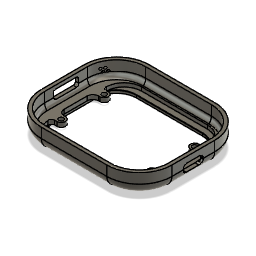
cube2025年6月14日 (Autodesk Fusion 360 design; units mm, degrees)
Autodesk Fusion 360 part; units mm, degrees
sketch "草图1" plane through (0, 0, 0) normal (0, 1, 0) x (1, 0, 0)
  line L0 (11.6, 15.075) -> (-11.6, 15.075)
  line L1 (-19.1, 7.575) -> (-19.1, -7.575)
  line L2 (-11.6, -15.075) -> (11.6, -15.075)
  line L3 (19.1, -7.575) -> (19.1, 7.575)
  line L4 (19.1, 15.075) -> (-19.1, -15.075) construction
  line L5 (-19.1, 15.075) -> (19.1, -15.075) construction
  arc A0 (-11.6, 15.075) -> (-19.1, 7.575) centre (-11.6, 7.575) ccw
  arc A1 (19.1, 7.575) -> (11.6, 15.075) centre (11.6, 7.575) ccw
  arc A2 (11.6, -15.075) -> (19.1, -7.575) centre (11.6, -7.575) ccw
  arc A3 (-19.1, -7.575) -> (-11.6, -15.075) centre (-11.6, -7.575) ccw
  dimension "d1" = 38.2
  dimension "d2" = 30.15
  dimension "d3" = 7.5
  dimension "d4" = 7.5
  constraint horizontal L0
  constraint perpendicular L0 L1
  constraint parallel L0 L2
  constraint parallel L1 L3
  constraint coincident L4 origin
  constraint coincident L5 origin
  constraint coincident L5.start L1
  constraint coincident L5.start L0
  constraint tangent L1 A0
  constraint tangent L0 A0
  constraint coincident L4.start L0
  constraint coincident L4.start L3
  constraint tangent L0 A1
  constraint tangent L3 A1
  constraint coincident L5.end L3
  constraint coincident L5.end L2
  constraint tangent L3 A2
  constraint tangent L2 A2
  constraint equal A1 A2
  constraint coincident L4.end L1
  constraint coincident L4.end L2
  constraint tangent L1 A3
  constraint tangent L2 A3
  constraint equal A1 A3
  measures "d1" distance of L4.end L5.end
  measures "d2" distance of L4.start L5.end
  measures "d3" radius of A0
  measures "d4" radius of A1
sketch "草图2" plane through (0, 0, 0) normal (0, 1, 0) x (1, 0, 0)
  circle A0 centre (17.3934, 13.5745) radius 0.65
  circle A1 centre (-17.3935, -13.5745) radius 0.65
  circle A2 centre (17.3934, -13.5745) radius 0.65
  circle A3 centre (-17.3935, 13.5745) radius 0.65
  arc A4 (-16.0995, 15.5745) -> (-19.3935, 12.4745) centre (-16.0995, 12.2745) ccw
  arc A5 (-19.3935, -12.4745) -> (-16.0995, -15.5745) centre (-16.0995, -12.2745) ccw
  arc A6 (16.0995, -15.5745) -> (19.3934, -12.4745) centre (16.0995, -12.2745) ccw
  line L0 (-16.0995, -15.5745) -> (16.0995, -15.5745)
  line L1 (19.3934, -12.4745) -> (19.3934, 12.4745)
  arc A7 (19.3934, 12.4745) -> (16.0995, 15.5745) centre (16.0995, 12.2745) ccw
  line L2 (-19.3935, 12.4745) -> (-19.3935, -12.4745)
  line L3 (16.0995, 15.5745) -> (-16.0995, 15.5745)
  line L4 (-17.3935, 13.5745) -> (17.3934, -13.5745)
  line L5 (17.3934, 13.5745) -> (-17.3935, -13.5745)
sketch "草图3" plane through (0, 0, 0) normal (0, 0, 1) x (1, 0, 0)
  line L0 (0, 0) -> (19.1, 0)
  line L1 (0, 0) -> (-19.1, 0)
  line L2 (0, 0) -> (0, 4.5)
  line L3 (0, 4.5) -> (23.1, 4.5)
  line L4 (0, 4.5) -> (-23.1, 4.5)
  line L5 (19.1, 0) -> (19.4, 0)
  line L6 (19.4, 0) -> (19.4, 0.5)
  line L7 (19.4, 0.5) -> (19.1, 0.5)
  line L8 (19.1, 0.5) -> (19.1, 0)
  line L9 (-19.1, 0) -> (-19.4, 0)
  line L10 (-19.4, 0) -> (-19.4, 0.5)
  line L11 (-19.4, 0.5) -> (-19.1, 0.5)
  line L12 (-19.1, 0.5) -> (-19.1, 0)
  circle A0 centre (19.1, 4.5) radius 4
  circle A1 centre (18.9017, 0.459) radius 0.5
  circle A2 centre (-19.1, 4.5) radius 4
  circle A3 centre (-18.9017, 0.459) radius 0.5
  circle A4 centre (19.1, 4.5) radius 2.8
  circle A5 centre (-19.1, 4.5) radius 2.8
  line L13 (0, 0) -> (0, 3)
  line L14 (0, 3) -> (21.5, 3)
  line L15 (0, 3) -> (-21.5, 3)
  dimension "d5" = 19.1
  dimension "d6" = 19.1
  dimension "d7" = 4.5
  dimension "d8" = 23.1
  dimension "d9" = 23.1
  dimension "d10" = 0.3
  dimension "d11" = 0.5
  dimension "d12" = 0.3
  dimension "d13" = 0.5
  dimension "d14" = 8
  dimension "d15" = 1
  dimension "d16" = 8
  dimension "d17" = 1
  dimension "d45" = 5.6
  dimension "d46" = 5.6
  dimension "d47" = 3
  constraint coincident L0.start L1.start
  constraint perpendicular L0 L2
  constraint perpendicular L2 L3
  constraint perpendicular L2 L4
  constraint horizontal L5
  constraint vertical L6
  constraint horizontal L7
  constraint vertical L8
  constraint horizontal L9
  constraint vertical L10
  constraint horizontal L11
  constraint vertical L12
  constraint coincident L7.end A0
  constraint coincident L3.end A0
  constraint coincident L0.end A1
  constraint coincident L6.end A1
  constraint coincident L4.end A2
  constraint coincident L11.end A2
  constraint coincident L10.end A3
  constraint coincident L1.end A3
  constraint concentric A0 A4
  constraint concentric A2 A5
  constraint perpendicular L0 L13
  constraint perpendicular L13 L14
  constraint perpendicular L2 L15
  measures "d5" distance of L0.start L0.end
  measures "d6" distance of L0.start L1.end
  measures "d7" distance of L0.start L2.end
  measures "d8" distance of L2.end L3.end
  measures "d9" distance of L2.end L4.end
  measures "d10" distance of L0.end L5.end
  measures "d11" distance of L0.end L7.end
  measures "d12" distance of L1.end L9.end
  measures "d13" distance of L9.end L10.end
  measures "d14" diameter of A0
  measures "d15" diameter of A1
  measures "d16" diameter of A2
  measures "d17" diameter of A3
  measures "d45" diameter of A4
  measures "d46" diameter of A5
  measures "d47" distance of L0.start L13.end
extrude "拉伸1" add sketch "草图3" along normal blind 7.575 contours L0 L2 A0 A1 L13 L14 | L1 L2 A2 A3 L13 L15 | L0 L8 A0 A1 | L0 A1 | L1 A3 | L1 L12 A2 A3 | L6 L7 L8 A1 | A0 A1 | L3 A0 A1 A4 L14 | L10 L11 L12 A3 | L4 A2 A3 A5 L15 | L7 A0 A1 | L11 A2 A3 | A2 A3 | A4 L14 | A5 L15 makes body 1
extrude "拉伸2" add 1 faces at (-11.3651, 1, 0) along direction (0, 0, -1) blind 7.575 on bodies 1 bodies 1
sketch "草图4" plane through (0, 0, 0) normal (1, 0, 0) x (0, 0, -1)
  line L0 (27, 17) -> (-34, 17)
  line L1 (-34, 17) -> (-34, -12)
  line L2 (-34, -12) -> (27, -12)
  line L3 (27, -12) -> (27, 17)
  constraint horizontal L0
  constraint vertical L1
  constraint horizontal L2
  constraint vertical L3
extrude "拉伸3" add sketch "草图4" along normal blind 11.6 bodies 1
sweep "扫掠1" add 1 faces at (13.9678, 1, -7.575) path "草图1" along A0 L1 A3 L2 A2 L3 A1 L0 on bodies 1 bodies 1
extrude "拉伸4" cut 1 faces at (11.6, 2.9679, 29.0101) along direction (-1, 0, 0) blind 17 on bodies 1 bodies 1
extrude "拉伸8" add 6 faces at (22.7, 4.5, 2.525) (3.8667, 4.5, -18.275) (3.8667, 4.5, 18.275) (-1.8, 4.5, -18.675) (-1.8, 4.5, 18.275) (-22.7, 4.5, 2.525) along direction (0, 1, 0) blind 3.5 separate body on bodies 1 makes body 2
extrude "拉伸9" cut 4 faces at (14.8881, 3, 2.525) (3.8667, 3, -5.8131) (-3.6, 3, 5.8131) (-10.7548, 3, -2.525) along direction (0, -1, 0) blind 0.5 on bodies 1 bodies 1
sketch "草图7" plane through (0, 0, 0) normal (0, -1, 0) x (1, 0, 0)
  arc A0 (11.6, -14.6784) -> (18.7034, -7.575) centre (11.6, -7.575) ccw
  line L0 (18.7034, -7.575) -> (18.7034, 7.575)
  arc A1 (18.7034, 7.575) -> (11.6, 14.6784) centre (11.6, 7.575) ccw
  line L1 (11.6, 14.6784) -> (-11.6, 14.6784)
  arc A2 (-11.6, 14.6784) -> (-18.7034, 7.575) centre (-11.6, 7.575) ccw
  line L2 (-18.7034, 7.575) -> (-18.7034, -7.575)
  arc A3 (-18.7034, -7.575) -> (-11.6, -14.6784) centre (-11.6, -7.575) ccw
  line L3 (-11.6, -14.6784) -> (11.6, -14.6784)
  line L4 (16, 7.575) -> (-16, 7.575)
  line L5 (-16, 7.575) -> (-16, -7.575)
  line L6 (-16, -7.575) -> (16, -7.575)
  line L7 (16, -7.575) -> (16, 7.575)
  line L8 (16, 7.575) -> (-16, -7.575) construction
  line L9 (-16, 7.575) -> (16, -7.575) construction
  line L10 (-11.6005, -14.4785) -> (11.6005, -14.4785)
  line L11 (18.5035, -4.075) -> (18.5035, 4.075)
  line L12 (11.6005, 14.4785) -> (-11.6005, 14.4785)
  line L13 (-18.5035, 4.075) -> (-18.5035, -4.075)
  line L14 (-18.5035, -14.4785) -> (18.5035, 14.4785) construction
  line L15 (18.5035, -14.4785) -> (-18.5035, 14.4785) construction
  arc A4 (11.6005, -14.4785) -> (17.8541, -10.4984) centre (11.6005, -7.5755) ccw
  arc A5 (-17.8541, -10.4984) -> (-11.6005, -14.4785) centre (-11.6005, -7.5755) ccw
  arc A6 (-11.6005, 14.4785) -> (-17.8541, 10.4984) centre (-11.6005, 7.5755) ccw
  arc A7 (17.8541, 10.4984) -> (11.6005, 14.4785) centre (11.6005, 7.5755) ccw
  circle A8 centre (16, -7.575) radius 1.5
  circle A9 centre (-16, -7.575) radius 1.5
  circle A10 centre (-16, 7.575) radius 1.5
  circle A11 centre (16, 7.575) radius 1.5
  line L16 (16, -7.575) -> (16, -9.075)
  line L17 (16, -9.075) -> (16.9482, -9.075)
  line L18 (14.5, -7.575) -> (14.5, 7.575)
  line L19 (16, 7.575) -> (16, 9.075)
  line L20 (16, 9.075) -> (16.9482, 9.075)
  line L21 (-16, -7.575) -> (-16, -9.075)
  line L22 (-16, -9.075) -> (-16.9482, -9.075)
  line L23 (-14.5, -7.575) -> (-14.5, 7.575)
  line L24 (-16, 7.575) -> (-16, 9.075)
  line L25 (-16, 9.075) -> (-16.9482, 9.075)
  arc A12 (17.8541, -10.4984) -> (16.9482, -9.075) centre (16.9482, -10.075) ccw
  arc A13 (16.9482, 9.075) -> (17.8541, 10.4984) centre (16.9482, 10.075) ccw
  arc A14 (-16.9482, -9.075) -> (-17.8541, -10.4984) centre (-16.9482, -10.075) ccw
  arc A15 (-17.8541, 10.4984) -> (-16.9482, 9.075) centre (-16.9482, 10.075) ccw
  line L26 (-16, -6.075) -> (-16.5035, -6.075)
  line L27 (-16, 6.075) -> (-16.5035, 6.075)
  arc A16 (-18.5035, -4.075) -> (-16.5035, -6.075) centre (-16.5035, -4.075) ccw
  arc A17 (-16.5035, 6.075) -> (-18.5035, 4.075) centre (-16.5035, 4.075) ccw
  line L28 (16, -6.075) -> (16.5035, -6.075)
  line L29 (16, 6.075) -> (16.5035, 6.075)
  arc A18 (18.5035, 4.075) -> (16.5035, 6.075) centre (16.5035, 4.075) ccw
  arc A19 (16.5035, -6.075) -> (18.5035, -4.075) centre (16.5035, -4.075) ccw
  dimension "d52" = 32
  dimension "d53" = 15.15
  dimension "d54" = 37.007
  dimension "d55" = 28.957
  dimension "d56" = 6.903
  dimension "d57" = 3
  dimension "d58" = 3
  dimension "d59" = 3
  dimension "d60" = 3
  dimension "d61" = 1
  dimension "d62" = 1
  dimension "d63" = 1
  dimension "d64" = 1
  dimension "d81" = 2
  dimension "d82" = 2
  dimension "d83" = 2
  dimension "d84" = 2
  constraint horizontal L4
  constraint perpendicular L4 L5
  constraint parallel L4 L6
  constraint parallel L5 L7
  constraint coincident L8 origin
  constraint coincident L9 origin
  constraint horizontal L10
  constraint perpendicular L10 L11
  constraint parallel L10 L12
  constraint parallel L11 L13
  constraint coincident L14 origin
  constraint coincident L15 origin
  constraint coincident L15.start L11
  constraint coincident L15.start L10
  constraint tangent L11 A4
  constraint tangent L10 A4
  constraint coincident L14.start L10
  constraint coincident L14.start L13
  constraint tangent L10 A5
  constraint tangent L13 A5
  constraint equal A4 A5
  constraint coincident L15.end L13
  constraint coincident L15.end L12
  constraint tangent L13 A6
  constraint tangent L12 A6
  constraint equal A4 A6
  constraint coincident L14.end L12
  constraint coincident L14.end L11
  constraint tangent L12 A7
  constraint tangent L11 A7
  constraint equal A4 A7
  constraint coincident L6.end L7.start
  constraint coincident L5.end L6.start
  constraint coincident L4.end L5.start
  constraint coincident L4.start L7.end
  constraint coincident A8 L16.end
  constraint perpendicular L6 L16
  constraint tangent A8 L17
  constraint coincident A8 L18.start
  constraint coincident L6 L18.start
  constraint coincident L4 L18.end
  constraint coincident A11 L18.end
  constraint coincident A11 L19.end
  constraint perpendicular L4 L19
  constraint tangent A11 L20
  constraint coincident A9 L21.end
  constraint perpendicular L6 L21
  constraint tangent A9 L22
  constraint coincident L6 L23.start
  constraint coincident A9 L23.start
  constraint coincident L4 L23.end
  constraint coincident A10 L23.end
  constraint coincident A10 L24.end
  constraint perpendicular L4 L24
  constraint tangent A10 L25
  constraint tangent A4 A12
  constraint tangent L17 A12
  constraint tangent L20 A13
  constraint tangent A7 A13
  constraint tangent A5 A14
  constraint tangent L22 A14
  constraint tangent L25 A15
  constraint tangent A6 A15
  constraint coincident A9 L26.start
  constraint coincident L5 L26.start
  constraint tangent A9 L26
  constraint coincident A10 L27.start
  constraint coincident L5 L27.start
  constraint tangent A10 L27
  constraint tangent L26 A16
  constraint tangent L13 A16
  constraint tangent L27 A17
  constraint tangent L13 A17
  constraint coincident A8 L28.start
  constraint coincident L7 L28.start
  constraint tangent A8 L28
  constraint coincident A11 L29.start
  constraint coincident L7 L29.start
  constraint tangent A11 L29
  constraint tangent L11 A18
  constraint tangent L29 A18
  constraint tangent L28 A19
  constraint tangent L11 A19
  measures "d52" distance of L5.end L6.end
  measures "d53" distance of L4.start L6.end
  measures "d54" distance of L14.end L15.end
  measures "d55" distance of L14.start L15.end
  measures "d56" radius of A4
  measures "d57" diameter of A8
  measures "d58" diameter of A9
  measures "d59" diameter of A10
  measures "d60" diameter of A11
  measures "d61" radius of A12
  measures "d62" radius of A13
  measures "d63" radius of A14
  measures "d64" radius of A15
  measures "d81" radius of A16
  measures "d82" radius of A17
  measures "d83" radius of A18
  measures "d84" radius of A19
extrude "拉伸10" cut 4 faces at (13.9678, 0, -2.525) (3.8667, 0, -4.8928) (-1.8, 0, 4.8928) (-9.8345, 0, -2.525) along direction (0, 1, 0) blind 1 on bodies 1 bodies 1
extrude "拉伸11" cut sketch "草图7" against normal blind 2.5 contours L4 L6 L18 L23 | L4 L12 A6 A7 A10 A11 L20 L25 A13 A15 | L7 A8 A11 L18 | L7 L11 L28 L29 A18 A19 | L5 A9 A10 L23 | L6 L10 A4 A5 A8 A9 L17 L22 A12 A14 | L5 L13 L26 L27 A16 A17 bodies 1
hole "孔1" at (-16, 0, -7.575) direction (0, 1, 0) diameter 1.7 depth 3.5 tip angle 180 bodies 1
hole "孔2" at (-16, 0, 7.575) direction (0, 1, 0) diameter 1.7 depth 3.5 tip angle 180 bodies 1
hole "孔3" at (16, 0, -7.575) direction (0, 1, 0) diameter 1.7 depth 3.5 tip angle 180 bodies 1
hole "孔4" at (16, 0, 7.575) direction (0, 1, 0) diameter 1.7 depth 3.5 tip angle 180 bodies 1
sketch "草图8" plane through (-23.1, 0, 0) normal (-1, 0, 0) x (0, 0, 1)
  line L0 (-7.575, 4.5) -> (7.575, 4.5)
  line L1 (7.575, 4.5) -> (7.575, 8)
  line L2 (7.575, 8) -> (-7.575, 8)
  line L3 (-7.575, 8) -> (-7.575, 4.5)
  line L4 (0, 0) -> (0, 3.6)
  line L5 (0, 3.6) -> (0, 5.23)
  line L6 (3.675, 3.7) -> (-3.675, 3.7)
  line L7 (-4.475, 4.5) -> (-4.475, 5.96)
  line L8 (-3.675, 6.76) -> (3.675, 6.76)
  line L9 (4.475, 5.96) -> (4.475, 4.5)
  line L10 (4.475, 3.7) -> (-4.475, 6.76) construction
  line L11 (-4.475, 3.7) -> (4.475, 6.76) construction
  arc A0 (4.475, 5.96) -> (3.675, 6.76) centre (3.675, 5.96) ccw
  arc A1 (3.675, 3.7) -> (4.475, 4.5) centre (3.675, 4.5) ccw
  arc A2 (-3.675, 6.76) -> (-4.475, 5.96) centre (-3.675, 5.96) ccw
  arc A3 (-4.475, 4.5) -> (-3.675, 3.7) centre (-3.675, 4.5) ccw
  point P0 (0, 5.23)
  dimension "d85" = 3.6
  dimension "d86" = 1.63
  dimension "d87" = 8.95
  dimension "d88" = 3.06
  dimension "d89" = 0.8
  constraint coincident L4.start origin
  constraint parallel L3 L4
  constraint perpendicular L0 L5
  constraint horizontal L6
  constraint perpendicular L6 L7
  constraint parallel L6 L8
  constraint parallel L7 L9
  constraint coincident L10 P0
  constraint coincident L11 P0
  constraint coincident P0 L5.end
  constraint coincident L11.end L8
  constraint coincident L11.end L9
  constraint tangent L8 A0
  constraint tangent L9 A0
  constraint coincident L10.start L9
  constraint coincident L10.start L6
  constraint tangent L9 A1
  constraint tangent L6 A1
  constraint equal A0 A1
  constraint coincident L10.end L8
  constraint coincident L10.end L7
  constraint tangent L8 A2
  constraint tangent L7 A2
  constraint equal A0 A2
  constraint coincident L11.start L7
  constraint coincident L11.start L6
  constraint tangent L7 A3
  constraint tangent L6 A3
  constraint equal A0 A3
  measures "d85" distance of L4.start L4.end
  measures "d86" distance of L4.end P0
  measures "d87" distance of L10.end L11.end
  measures "d88" distance of L10.start L11.end
  measures "d89" radius of A0
extrude "拉伸12" cut sketch "草图8" against normal blind 5 contours L0 L7 L8 L9 A0 A2 | L0 L5 L6 A3 | L0 L5 L6 A1 bodies 1 2
sketch "草图9" plane through (23.1, 0, 0) normal (1, 0, 0) x (0, 0, -1)
  line L0 (-7.575, 4.5) -> (7.575, 4.5)
  line L1 (7.575, 4.5) -> (7.575, 8)
  line L2 (7.575, 8) -> (-7.575, 8)
  line L3 (-7.575, 8) -> (-7.575, 4.5)
  line L4 (0, 0) -> (0, 3.6)
  line L5 (0, 3.6) -> (0, 4.45)
  line L6 (2.25, 2.95) -> (-2.25, 2.95)
  line L7 (-3.5, 4.2) -> (-3.5, 4.7)
  line L8 (-2.25, 5.95) -> (2.25, 5.95)
  line L9 (3.5, 4.7) -> (3.5, 4.2)
  line L10 (3.5, 2.95) -> (-3.5, 5.95) construction
  line L11 (-3.5, 2.95) -> (3.5, 5.95) construction
  arc A0 (3.5, 4.7) -> (2.25, 5.95) centre (2.25, 4.7) ccw
  arc A1 (2.25, 2.95) -> (3.5, 4.2) centre (2.25, 4.2) ccw
  arc A2 (-3.5, 4.2) -> (-2.25, 2.95) centre (-2.25, 4.2) ccw
  arc A3 (-2.25, 5.95) -> (-3.5, 4.7) centre (-2.25, 4.7) ccw
  point P0 (0, 4.45)
  dimension "d92" = 3.6
  dimension "d93" = 0.85
  dimension "d94" = 7
  dimension "d95" = 3
  dimension "d96" = 1.25
  dimension "d97" = 1.25
  constraint coincident L4.start origin
  constraint perpendicular L0 L4
  constraint perpendicular L0 L5
  constraint horizontal L6
  constraint perpendicular L6 L7
  constraint parallel L6 L8
  constraint parallel L7 L9
  constraint coincident L10 P0
  constraint coincident L11 P0
  constraint coincident P0 L5.end
  constraint coincident L11.end L8
  constraint coincident L11.end L9
  constraint tangent L8 A0
  constraint tangent L9 A0
  constraint coincident L10.start L9
  constraint coincident L10.start L6
  constraint tangent L9 A1
  constraint tangent L6 A1
  constraint coincident L11.start L6
  constraint coincident L11.start L7
  constraint tangent L6 A2
  constraint tangent L7 A2
  constraint equal A1 A2
  constraint coincident L10.end L8
  constraint coincident L10.end L7
  constraint tangent L8 A3
  constraint tangent L7 A3
  constraint equal A1 A3
  measures "d92" distance of L4.start L4.end
  measures "d93" distance of L4.end P0
  measures "d94" distance of L10.end L11.end
  measures "d95" distance of L10.start L11.end
  measures "d96" radius of A0
  measures "d97" radius of A1
extrude "拉伸13" cut sketch "草图9" against normal blind 5 contours L0 L7 L8 L9 A0 A3 | L0 L6 L7 L9 A1 A2 bodies 1 2
sketch "草图10" plane through (0, 0, 0) normal (1, 0, 0) x (0, 0, -1)
  line L0 (0, 0) -> (0, 3.6)
  line L1 (0, 3.6) -> (0, 4.45)
  line L2 (4.205, 3.2) -> (-4.205, 3.2)
  line L3 (-4.805, 3.8) -> (-4.805, 5.1)
  line L4 (-4.205, 5.7) -> (4.205, 5.7)
  line L5 (4.805, 5.1) -> (4.805, 3.8)
  line L6 (4.805, 3.2) -> (-4.805, 5.7) construction
  line L7 (-4.805, 3.2) -> (4.805, 5.7) construction
  arc A0 (4.805, 5.1) -> (4.205, 5.7) centre (4.205, 5.1) ccw
  arc A1 (4.205, 3.2) -> (4.805, 3.8) centre (4.205, 3.8) ccw
  arc A2 (-4.805, 3.8) -> (-4.205, 3.2) centre (-4.205, 3.8) ccw
  arc A3 (-4.205, 5.7) -> (-4.805, 5.1) centre (-4.205, 5.1) ccw
  point P0 (0, 4.45)
  dimension "d100" = 3.6
  dimension "d101" = 0.85
  dimension "d102" = 9.61
  dimension "d103" = 2.5
  dimension "d104" = 0.6
  constraint coincident L0.start origin
  constraint vertical L0
  constraint parallel L0 L1
  constraint horizontal L2
  constraint perpendicular L2 L3
  constraint parallel L2 L4
  constraint parallel L3 L5
  constraint coincident L6 P0
  constraint coincident L7 P0
  constraint coincident P0 L1.end
  constraint coincident L7.end L4
  constraint coincident L7.end L5
  constraint tangent L4 A0
  constraint tangent L5 A0
  constraint coincident L6.start L5
  constraint coincident L6.start L2
  constraint tangent L5 A1
  constraint tangent L2 A1
  constraint equal A0 A1
  constraint coincident L7.start L2
  constraint coincident L7.start L3
  constraint tangent L2 A2
  constraint tangent L3 A2
  constraint equal A0 A2
  constraint coincident L6.end L4
  constraint coincident L6.end L3
  constraint tangent L4 A3
  constraint tangent L3 A3
  constraint equal A0 A3
  measures "d100" distance of L0.start L0.end
  measures "d101" distance of L0.end P0
  measures "d102" distance of L6.end L7.end
  measures "d103" distance of L6.start L7.end
  measures "d104" radius of A0
extrude "拉伸14" cut sketch "草图10" along normal blind 22.2 bodies 1 2
sketch "草图11" plane through (0, 2.5, 0) normal (0, 1, 0) x (-1, 0, 0)
  circle A0 centre (-16, 7.575) radius 0.85
  circle A1 centre (-16, -7.575) radius 0.85
  circle A2 centre (16, 7.575) radius 0.85
  circle A3 centre (16, -7.575) radius 0.85
  arc A4 (-18.5035, -4.075) -> (-16.5035, -6.075) centre (-16.5035, -4.075) ccw
  line L0 (-18.5035, -4.075) -> (-18.5035, 4.075)
  arc A5 (-16.5035, 6.075) -> (-18.5035, 4.075) centre (-16.5035, 4.075) ccw
  line L1 (-16.5035, 6.075) -> (-16, 6.075)
  arc A6 (-16, 6.075) -> (-16, 9.075) centre (-16, 7.575) ccw
  line L2 (-16, 9.075) -> (-16.9482, 9.075)
  arc A7 (-17.8541, 10.4984) -> (-16.9482, 9.075) centre (-16.9482, 10.075) ccw
  arc A8 (-11.6005, 14.4785) -> (-17.8541, 10.4984) centre (-11.6005, 7.5755) ccw
  line L3 (-11.6005, 14.4785) -> (11.6005, 14.4785)
  arc A9 (17.8541, 10.4984) -> (11.6005, 14.4785) centre (11.6005, 7.5755) ccw
  arc A10 (16.9482, 9.075) -> (17.8541, 10.4984) centre (16.9482, 10.075) ccw
  line L4 (16.9482, 9.075) -> (16, 9.075)
  arc A11 (16, 9.075) -> (16, 6.075) centre (16, 7.575) ccw
  line L5 (16, 6.075) -> (16.5035, 6.075)
  arc A12 (18.5035, 4.075) -> (16.5035, 6.075) centre (16.5035, 4.075) ccw
  line L6 (18.5035, 4.075) -> (18.5035, -4.075)
  arc A13 (16.5035, -6.075) -> (18.5035, -4.075) centre (16.5035, -4.075) ccw
  line L7 (16.5035, -6.075) -> (16, -6.075)
  arc A14 (16, -6.075) -> (16, -9.075) centre (16, -7.575) ccw
  line L8 (16, -9.075) -> (16.9482, -9.075)
  arc A15 (17.8541, -10.4984) -> (16.9482, -9.075) centre (16.9482, -10.075) ccw
  arc A16 (11.6005, -14.4785) -> (17.8541, -10.4984) centre (11.6005, -7.5755) ccw
  line L9 (11.6005, -14.4785) -> (-11.6005, -14.4785)
  arc A17 (-17.8541, -10.4984) -> (-11.6005, -14.4785) centre (-11.6005, -7.5755) ccw
  arc A18 (-16.9482, -9.075) -> (-17.8541, -10.4984) centre (-16.9482, -10.075) ccw
  line L10 (-16.9482, -9.075) -> (-16, -9.075)
  arc A19 (-16, -9.075) -> (-16, -6.075) centre (-16, -7.575) ccw
  line L11 (-16, -6.075) -> (-16.5035, -6.075)
  arc A20 (-11.6, 17.4393) -> (-21.4643, 7.575) centre (-11.6, 7.575) ccw
  line L12 (-21.4643, 7.575) -> (-21.4643, -7.575)
  arc A21 (-21.4643, -7.575) -> (-11.6, -17.4393) centre (-11.6, -7.575) ccw
  line L13 (-11.6, -17.4393) -> (11.6, -17.4393)
  arc A22 (11.6, -17.4393) -> (21.4643, -7.575) centre (11.6, -7.575) ccw
  line L14 (21.4643, -7.575) -> (21.4643, 7.575)
  arc A23 (21.4643, 7.575) -> (11.6, 17.4393) centre (11.6, 7.575) ccw
  line L15 (11.6, 17.4393) -> (-11.6, 17.4393)
  line L16 (-11.6005, -16.48) -> (11.6005, -16.48)
  line L17 (11.6005, -16.48) -> (11.6005, 16.48)
  line L18 (11.6005, 16.48) -> (-11.6005, 16.48)
  line L19 (-11.6005, 16.48) -> (-11.6005, -16.48)
  line L20 (-11.6005, -16.48) -> (11.6005, 16.48) construction
  line L21 (11.6005, -16.48) -> (-11.6005, 16.48) construction
  circle A24 centre (-11.6005, -10.18) radius 6.3
  circle A25 centre (11.6005, -10.18) radius 6.3
  circle A26 centre (-11.6005, 10.18) radius 6.3
  circle A27 centre (11.6005, 10.18) radius 6.3
  dimension "d107" = 32.96
  dimension "d108" = 23.201
  dimension "d109" = 12.6
  dimension "d110" = 12.6
  dimension "d111" = 12.6
  dimension "d112" = 12.6
  constraint horizontal L16
  constraint perpendicular L16 L17
  constraint parallel L16 L18
  constraint parallel L17 L19
  constraint coincident L20 origin
  constraint coincident L21 origin
  constraint tangent L16 A24
  constraint coincident L19 A24.centre
  constraint tangent L16 A25
  constraint tangent L18 A27
  constraint tangent L18 A26
  constraint coincident L19 A26.centre
  constraint coincident L17 A27.centre
  constraint coincident L17 A25.centre
  measures "d107" distance of L16.start L18.end
  measures "d108" distance of L16.start L16.end
  measures "d109" diameter of A24
  measures "d110" diameter of A25
  measures "d111" diameter of A26
  measures "d112" diameter of A27
extrude "拉伸15" cut sketch "草图11" against normal blind 1.3 contours A17 A18 L19 A24 | L9 L19 A24 | L3 L19 A26 | A7 A8 L19 A26 | L9 L16 A24 A25 | L3 L18 A26 A27 | L9 L17 A25 | A15 A16 L17 A25 | L3 L17 A27 | A9 A10 L17 A27 picked at (-11.3144, -15.7933) picked at (-11.3144, 15.7933) picked at (11.3144, -15.7933) picked at (11.3144, 15.7933) bodies 1
delete_face "删除面1" 12 faces at (7.7333, 2.8333, 17.4393) (-3.6, 2.8333, 17.4393) (-9.5333, 2.8333, 17.4393) (-12.0694, 2.6667, 17.4281) (-21.4643, 2.6667, -2.525) (-21.4531, 2.6667, -8.0444) (7.7333, 2.6667, -17.4393) (-1.8, 2.8333, -17.4393) (-7.4667, 2.8333, -17.4393) (21.1863, 2.6667, -9.9006) (21.4643, 2.8333, 5.9167) (17.6977, 2.6667, 15.3289) on bodies 1
sketch "草图14" plane through (-23.1, 0, 0) normal (-1, 0, 0) x (0, 0, 1)
  line L0 (-4.475, 4.5) -> (-4.475, 5.96)
  arc A0 (-3.675, 6.76) -> (-4.475, 5.96) centre (-3.675, 5.96) ccw
  line L1 (-3.675, 6.76) -> (3.675, 6.76)
  arc A1 (4.475, 5.96) -> (3.675, 6.76) centre (3.675, 5.96) ccw
  line L2 (4.475, 5.96) -> (4.475, 4.5)
  line L3 (4.475, 4.5) -> (7.575, 4.5)
  line L4 (7.575, 4.5) -> (7.575, 8)
  line L5 (7.575, 8) -> (-7.575, 8)
  line L6 (-7.575, 8) -> (-7.575, 4.5)
  line L7 (-7.575, 4.5) -> (-4.475, 4.5)
  circle A2 centre (-13.2, 4.8) radius 0.4
  circle A3 centre (-12, 4.8) radius 0.4
  circle A4 centre (-12.6, 5.8392) radius 0.4
  circle A5 centre (-11.4, 5.8392) radius 0.4
  line L8 (0, 0) -> (-12, 0)
  line L9 (-12, 0) -> (-12, 4.8)
  line L10 (-12.6, 5.8392) -> (-12, 4.8)
  line L11 (-12, 4.8) -> (-11.4, 5.8392)
  line L12 (-11.4, 5.8392) -> (-12.6, 5.8392)
  line L13 (-13.2, 4.8) -> (-12.6, 5.8392)
  line L14 (-13.2, 4.8) -> (-12, 4.8)
  dimension "d120" = 0.8
  dimension "d121" = 0.8
  dimension "d122" = 0.8
  dimension "d123" = 0.8
  dimension "d124" = 12
  dimension "d125" = 4.8
  dimension "d126" = 1.2
  constraint coincident L8.start origin
  constraint horizontal L8
  constraint perpendicular L8 L9
  constraint coincident A4.centre L10.start
  constraint coincident A3.centre L9.end
  constraint coincident A5.centre L11.end
  constraint coincident A2.centre L13.start
  constraint equal L11 L12
  constraint equal L10 L11
  constraint equal L11 L13
  constraint equal L11 L14
  constraint parallel L8 L14
  measures "d120" diameter of A2
  measures "d121" diameter of A3
  measures "d122" diameter of A4
  measures "d123" diameter of A5
  measures "d124" distance of L8.start L8.end
  measures "d125" distance of L8.end A3.centre
  measures "d126" distance of A3.centre A5.centre
extrude "拉伸16" cut sketch "草图14" against normal blind 5.5 contours A2 L13 L14 | A2 L13 L14 | A3 L9 L14 | A3 L10 L14 | A4 L10 L13 | A4 L12 L13 | A3 L10 L11 | A3 L9 L11 | A4 L10 L12 | A5 L11 L12 | A5 L11 L12 bodies 1 2
